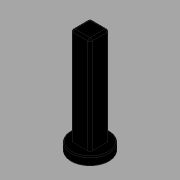
# Autodesk Inventor part: AXp2c
Saved by Autodesk Inventor 2019.3 (Build 233278000, 278)
## iProperties
Company: Unknown
Created: 2018-11-05
Part Number: AXp2c
Material: Generic
Description: Unknown
Document SubType Name: Modeling
Designer: Varga Daniel
Density: 1 g/cm^3
Appearance: Default
Mass: 0.340899 g
Surface Area: 3.95903 cm^2
Volume: 0.340899 cm^3
Sending System: DEX
Preprocessor: ST-DEVELOPER v16.7
Axle_length: 20,000 mm
Upper_fillet: 0,400 mm
Title: Axeis 2
Author: Unknown
Autodesk Inventor part; units mm, degrees
ref_plane "YZ Plane" through (0, 0, 0) normal (1, 0, 0) x (0, 1, 0)
ref_plane "XZ Plane" through (0, 0, 0) normal (0, 1, 0) x (-1, 0, 0)
ref_plane "XY Plane" through (0, 0, 0) normal (0, 0, 1) x (1, 0, 0)
derived "Connector_pin_base.ipt"
sketch "Pin_base_sketch" plane through (0, 0, 0) normal (0, 0, 1) x (1, 0, 0)
  line L0 (0, 0) -> (23.0918, 0) construction
  line L1 (0, 0) -> (0, 6.22) construction
  line L2 (0, 3.75) -> (0.55, 3.75)
  line L3 (0.85, 3.45) -> (0.85, 2.5)
  line L4 (0.85, 2.5) -> (10, 2.5)
  line L5 (10, 2.5) -> (10, 0)
  line L6 (0, 0) -> (0, 3.75)
  line L7 (0, 0) -> (10, 0)
  line L8 (9.25, 2.5) -> (9.25, 2.625)
  line L9 (10, 2.5) -> (10, 2.5024)
  arc A0 (10, 2.5024) -> (9.9256, 2.6604) centre (9.795, 2.5024) ccw
  arc A1 (9.9256, 2.6604) -> (9.25, 2.625) centre (9.6071, 2.275) ccw
  line L10 (9.9256, 2.6604) -> (9.9256, -0.0789) construction
  line L11 (8.9584, 2.775) -> (10.3858, 2.775) construction
  arc A2 (0.85, 3.45) -> (0.55, 3.75) centre (0.55, 3.45) ccw
  line L12 (0.85, 2.5) -> (0.85, 0)
  line L13 (-0.85, 2.5) -> (-0.85, 0)
  line L14 (-0.85, 3.45) -> (-0.85, 2.5)
  arc A3 (-0.55, 3.75) -> (-0.85, 3.45) centre (-0.55, 3.45) ccw
  line L15 (0, 3.75) -> (-0.55, 3.75)
  line L16 (0, 0) -> (-23.0918, 0) construction
  line L17 (0, 0) -> (-10, 0)
  line L18 (-0.85, 2.5) -> (-10, 2.5)
  line L19 (-9.25, 2.5) -> (-9.25, 2.625)
  arc A4 (-9.25, 2.625) -> (-9.9256, 2.6604) centre (-9.6071, 2.275) ccw
  arc A5 (-9.9256, 2.6604) -> (-10, 2.5024) centre (-9.795, 2.5024) ccw
  line L20 (-10, 2.5) -> (-10, 2.5024)
  line L21 (-8.9584, 2.775) -> (-10.3858, 2.775) construction
  line L22 (-9.9256, 2.6604) -> (-9.9256, -0.0789) construction
  line L23 (-10, 2.5) -> (-10, 0)
  line L24 (9.625, 3.2563) -> (9.625, -1.1868) construction
  dimension "d31" = 1.7
  measures "d31" distance between parallel lines of L13 L12
derived "Base_part.ipt"
sketch "Axle_sketch" plane through (0, 0, 0) normal (0, 1, 0) x (-1, 0, 0)
  circle A0 centre (-15.8957, 4.3197) radius 2.5 construction
  line L0 (-14.4207, 2.4447) -> (-17.3707, 2.4447)
  line L1 (-17.7707, 2.8447) -> (-17.7707, 5.7947)
  line L2 (-17.3707, 6.1947) -> (-14.4207, 6.1947)
  line L3 (-14.0207, 5.7947) -> (-14.0207, 2.8447)
  line L4 (-14.0207, 2.4447) -> (-17.7707, 6.1947) construction
  line L5 (-17.7707, 2.4447) -> (-14.0207, 6.1947) construction
  arc A1 (-14.4207, 2.4447) -> (-14.0207, 2.8447) centre (-14.4207, 2.8447) ccw
  arc A2 (-17.7707, 2.8447) -> (-17.3707, 2.4447) centre (-17.3707, 2.8447) ccw
  arc A3 (-14.0207, 5.7947) -> (-14.4207, 6.1947) centre (-14.4207, 5.7947) ccw
  arc A4 (-17.3707, 6.1947) -> (-17.7707, 5.7947) centre (-17.3707, 5.7947) ccw
  point P0 (0, 0)
sketch "Sketch1" plane through (0, 0, 0) normal (0, 1, 0) x (-1, 0, 0)
  line L0 (-1.475, -1.875) -> (1.475, -1.875)
  line L1 (1.875, -1.475) -> (1.875, 1.475)
  line L2 (1.475, 1.875) -> (-1.475, 1.875)
  line L3 (-1.875, 1.475) -> (-1.875, -1.475)
  line L4 (-1.875, -1.875) -> (1.875, 1.875) construction
  line L5 (1.875, -1.875) -> (-1.875, 1.875) construction
  arc A0 (-1.875, -1.475) -> (-1.475, -1.875) centre (-1.475, -1.475) ccw
  arc A1 (1.475, -1.875) -> (1.875, -1.475) centre (1.475, -1.475) ccw
  arc A2 (1.875, 1.475) -> (1.475, 1.875) centre (1.475, 1.475) ccw
  arc A3 (-1.475, 1.875) -> (-1.875, 1.475) centre (-1.475, 1.475) ccw
  circle A4 centre (0, 0) radius 2.5 construction
  line L6 (-14.4207, 2.4447) -> (-17.3707, 2.4447) construction
  arc A5 (-14.4207, 2.4447) -> (-14.0207, 2.8447) centre (-14.4207, 2.8447) ccw construction
  line L7 (-14.0207, 5.7947) -> (-14.0207, 2.8447) construction
  circle A6 centre (-15.8957, 4.3197) radius 2.5 construction
  line L8 (-17.3707, 6.1947) -> (-14.4207, 6.1947) construction
  arc A7 (-17.3707, 6.1947) -> (-17.7707, 5.7947) centre (-17.3707, 5.7947) ccw construction
  line L9 (-17.7707, 2.8447) -> (-17.7707, 5.7947) construction
  arc A8 (-17.7707, 2.8447) -> (-17.3707, 2.4447) centre (-17.3707, 2.8447) ccw construction
  arc A9 (-14.0207, 5.7947) -> (-14.4207, 6.1947) centre (-14.4207, 5.7947) ccw construction
  dimension "d0" = 3.75
  dimension "d1" = 3.75
  dimension "d2" = 0.4
  dimension "d11" = 5
  dimension "d13" = 3.75
  dimension "d14" = 0.4
  constraints: 12 end point, 8 point on circle, 8 point on line, 8 tangent, 5 centre point, 3 equal radius, 2 midpoint, 2 parallel, 1 coincident, 1 horizontal, 1 perpendicular
  measures "d0" distance of L4.end L5.end
  measures "d1" distance between parallel lines of L2 L0
  measures "d2" radius of A0
  measures "d11" diameter of A4
  measures "d13" distance between parallel lines of L7 L9
  measures "d14" radius of A8
extrude "Extrusion4" add sketch "Sketch1" along normal blind 19.15
fillet "Fillet2" radius 0.4 8 edges at (1.7578, 19.15, -1.7578) (0, 19.15, -1.875) (-1.7578, 19.15, -1.7578) (-1.875, 19.15, 0) (-1.7578, 19.15, 1.7578) (0, 19.15, 1.875) (1.7578, 19.15, 1.7578) (1.875, 19.15, 0)
ref_plane "Work Plane3" through (-1.475, 0, 0) normal (0, 0, 1) x (1, 0, 0)
ref_plane "Work Plane4" through (0, 0, -1.475) normal (-1, 0, 0) x (0, 0, 1)
sketch "Sketch6" plane through (0, 0, 0) normal (0, 0, 1) x (1, 0, 0)
  line L0 (0.85, 2.5) -> (0.85, 0) construction
  line L1 (0.85, 3.45) -> (0.85, 2.5) construction
  arc A0 (0.85, 3.45) -> (0.55, 3.75) centre (0.55, 3.45) ccw construction
  line L2 (0, 3.75) -> (0.55, 3.75) construction
  line L3 (0, 0) -> (0, 6.22) construction
  line L4 (0, 0) -> (23.0918, 0) construction
  line L5 (-1.475, 0) -> (1.475, 0) construction
  line L6 (-1.875, 0) -> (-1.875, 18.75) construction
  line L7 (1.875, 0) -> (1.875, 18.75) construction
  line L8 (1.475, 0) -> (-1.475, 0) construction
  line L9 (1.875, 0) -> (1.475, 0) construction
  line L10 (1.475, 0) -> (1.875, 0) construction
  line L11 (-1.475, 0) -> (1.475, 0) construction
  line L12 (-1.875, 0) -> (-1.475, 0) construction
  line L13 (-1.475, 0) -> (-1.875, 0) construction
  line L14 (0, 0) -> (0, -2.3465) construction
  line L15 (0, 34.9693) -> (0, -8.5658) construction
  line L16 (0, 0) -> (3.55, 0)
  line L17 (0, -1.7) -> (3.55, -1.7)
  line L18 (3.75, -1.5) -> (3.75, -0.2)
  arc A1 (3.75, -0.2) -> (3.55, 0) centre (3.55, -0.2) ccw
  arc A2 (3.55, -1.7) -> (3.75, -1.5) centre (3.55, -1.5) ccw
  line L19 (0, -1.7) -> (0, 0)
  dimension "d19" = 7.5
  dimension "d20" = 0.3
  dimension "d21" = 7.5
  dimension "d23" = 1.7
  dimension "d24" = 0.2
  dimension "d25" = 0.2
  constraints: 10 end point, 4 point on circle, 4 tangent, 2 centre point, 2 collinear, 2 point on line, 1 horizontal, 1 perpendicular
  measures "d19" diameter of L2 L4
  measures "d20" radius of A0
  measures "d21" diameter of L18 L14
  measures "d23" distance between parallel lines of L17 L16
  measures "d24" radius of A1
  measures "d25" radius of A2
revolve "Revolution1" add sketch "Sketch6" angle 360 about axis through (0, 0, 0) along (0, 1, 0)
fillet "Fillet3" [suppressed]
sketch "Sketch7" plane through (1.875, 18.75, 1.475) normal (1, 0, 0) x (0, 0, -1)
  line L0 (2.95, -18.75) -> (2.95, 0) projected
  line L1 (0, 0) -> (2.95, 0) projected
  line L2 (0, -18.75) -> (0, 0) projected
  line L3 (12.95, 10) -> (12.95, -29.4)
  line L4 (12.95, -29.4) -> (-10, -29.4)
  line L5 (-10, -29.4) -> (-10, 10)
  line L6 (-10, 10) -> (12.95, 10)
  line L7 (0, -18.75) -> (2.95, -18.75) projected
  point P0 (1.475, -18.75)
  dimension "d28" = 10
  constraints: 8 end point, 1 other
  measures "d28" distance between parallel lines of L0 L3
extrude "Printable_extrusion" [suppressed]
equation "\"d0\" = d13"
equation "\"d1\" = d0"
equation "\"d2\" = d14"
equation "\"d15\" = Axle_length - 0.5 * d31"
equation "\"d17\" = Upper_fillet"
equation "\"d21\" = d19"
equation "\"d23\" = d31"
equation "\"d24\" = Axle_collar_fillet"
equation "\"d25\" = d24"
equation "\"d27\" = Axle_collar_fillet"
equation "\"Axle_length\" = 20"
equation "\"Upper_fillet\" = 0.4"
equation "\"Axle_collar_fillet\" = 0.2"
equation "\"Axle_collar_thickness\" = 1.8"
body "Solid1"
